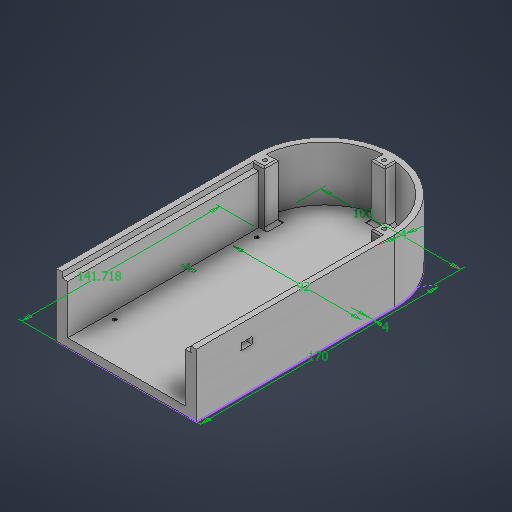
# Autodesk Inventor part: BASE_MANIPULADOR
Saved by Autodesk Inventor 2027.1 (Build 311270010, 270A)
## iProperties
Created: 2026-08-16
Part Number: BASE_MANIPULADOR
Material: Genérico
Document SubType Name: Modeling
Designer: Evellyn
Density: 1 g/cm^3
Appearance: Padrão
Author: Evellyn
Autodesk Inventor part; units mm, degrees
ref_plane "YZ Plane" through (0, 0, 0) normal (1, 0, 0) x (0, 1, 0)
ref_plane "XZ Plane" through (0, 0, 0) normal (0, 1, 0) x (-1, 0, 0)
ref_plane "XY Plane" through (0, 0, 0) normal (0, 0, 1) x (1, 0, 0)
sketch "Esboço1" plane through (0, 0, 0) normal (0, 1, 0) x (-1, 0, 0)
  point P0 (0, 0)
sketch "Esboço2" plane through (0, 0, 0) normal (0, 1, 0) x (-1, 0, 0)
  line L0 (50, -56.7182) -> (50, 85)
  line L1 (50, 85) -> (-50, 85)
  line L2 (-50, 85) -> (-50, -56.7182)
  line L3 (-50, -85) -> (50, 85) construction
  line L4 (50, -85) -> (-50, 85) construction
  line L5 (50, 0) -> (-50, 0)
  line L6 (-50, 0) -> (-50, -56.7182)
  line L7 (50, -56.7182) -> (50, 0)
  line L8 (0, 0) -> (0, -6.7182)
  arc A0 (-50, -56.7182) -> (50, -56.7182) centre (0, -56.7182) ccw
  line L9 (46, 85) -> (46, -56.7182)
  line L10 (-46, 85.0696) -> (-46, -56.7182)
  arc A1 (-46, -56.7182) -> (46, -56.7182) centre (0, -56.7182) ccw
  point P0 (-46, 85)
  dimension "d0" = 170
  dimension "d1" = 100
  dimension "d2" = 4
  dimension "d64" = 141.7182
  dimension "d70" = 4
  dimension "d71" = 4
  dimension "d72" = 92
  constraints: 22 end point, 5 point on circle, 3 point on line, 2 centre point, 2 midpoint, 2 parallel, 1 concentric, 1 horizontal, 1 perpendicular, 1 tangent, 1 vertical
  measures "d0" distance of L1.end L3.start
  measures "d1" distance of L3.start L4.start
  measures "d2" distance between parallel lines of L9 L0
  measures "d64" distance of L0.start L0.end
  measures "d70" distance between parallel lines of L6 L10
  measures "d71" radial gap between concentric circles of A1 A0
  measures "d72" distance between parallel lines of L10 L9
extrude "Extrusão3" add sketch "Esboço2" along normal blind 6 contours L9 A1 L10 L5 | L5 L10 L1 L9
extrude "Extrusão4" add sketch "Esboço2" along normal blind 45 contours A0 L2 L5 L10 A1 L9 L0 | L5 L9 L1 L0 | L2 L1 L10 L5
sketch "Esboço3" plane through (0, 6, 0) normal (0, 1, 0) x (1, 0, 0)
  line L0 (-37.999, -80.9605) -> (38.001, -80.9605)
  line L1 (40.001, -78.9605) -> (40.001, 62.0395)
  line L2 (38.001, 64.0395) -> (-37.999, 64.0395)
  line L3 (-39.999, 62.0395) -> (-39.999, -78.9605)
  line L4 (-46, -85) -> (-46, 56.7182) projected
  arc A0 (-39.999, -78.9605) -> (-37.999, -80.9605) centre (-37.999, -78.9605) ccw
  arc A1 (-37.999, 64.0395) -> (-39.999, 62.0395) centre (-37.999, 62.0395) ccw
  arc A2 (-37.999, 64.0395) -> (-39.999, 62.0395) centre (-37.999, 62.0395) ccw
  arc A3 (38.001, -80.9605) -> (40.001, -78.9605) centre (38.001, -78.9605) ccw
  circle A4 centre (-36.649, -56.8397) radius 1.35
  circle A5 centre (36.651, -56.7985) radius 1.35
  circle A6 centre (-36.649, 44.8205) radius 1.35
  circle A7 centre (36.651, 44.8205) radius 1.35
  arc A8 (40.001, 62.0395) -> (38.001, 64.0395) centre (38.001, 62.0395) ccw
  point P0 (0, 0)
  point P1 (40.001, 64.0395)
  point P2 (40.001, -80.9605)
  point P3 (-39.999, 64.0395)
  dimension "d11" = 80
  dimension "d12" = 145
  dimension "d13" = 6.001
  dimension "d14" = 2
  dimension "d15" = 2.7
  dimension "d17" = 3.35
  dimension "d18" = 2.7
  dimension "d19" = 3.35
  dimension "d20" = 22.162
  dimension "d21" = 2.7
  dimension "d22" = 3.35
  dimension "d23" = 17.219
  dimension "d24" = 2.7
  dimension "d25" = 3.35
  dimension "d26" = 2
  dimension "d27" = 17.219
  constraints: 10 point on circle, 10 tangent, 9 centre point, 8 end point, 8 point on line, 3 equal radius, 2 parallel, 1 horizontal, 1 perpendicular
  measures "d11" distance of point (-39.999, 64.039) point (40.001, 64.039)
  measures "d12" distance of point (40.001, 64.039) point (40.001, -80.961)
  measures "d13" distance between parallel lines of L4 L3
  measures "d14" radius of A0
  measures "d15" diameter of A4
  measures "d17" distance from line of L3 A4.centre
  measures "d18" diameter of A5
  measures "d19" distance from line of L1 A5.centre
  measures "d20" vertical distance of A5.centre A3.centre
  measures "d21" diameter of A6
  measures "d22" distance from line of L3 A6.centre
  measures "d23" vertical distance of A2.centre A6.centre
  measures "d24" diameter of A7
  measures "d25" distance from line of L1 A7.centre
  measures "d26" radius of A8
  measures "d27" vertical distance of A8.centre A7.centre
extrude "Extrusão5" cut sketch "Esboço3" against normal blind 3 contours A4 | A5 | A6 | A7
sketch "Esboço4" plane through (0, 6, 0) normal (0, 1, 0) x (1, 0, 0)
  arc A0 (46, 56.7182) -> (-46, 56.7182) centre (0, 56.7182) ccw projected
  line L0 (-46, -85) -> (-46, 56.7182) projected
  line L1 (46, 56.7182) -> (46, -85) projected
  line L2 (0, 112.992) -> (0, 0)
  line L3 (-5, 94.9519) -> (5, 94.9519)
  line L4 (5, 94.9519) -> (5, 104.9519)
  line L5 (5, 104.9519) -> (-5, 104.9519)
  line L6 (-5, 104.9519) -> (-5, 94.9519)
  line L7 (-5, 94.9519) -> (5, 104.9519) construction
  line L8 (5, 94.9519) -> (-5, 104.9519) construction
  circle A1 centre (0, 56.7182) radius 48.2336
  arc A2 (50, 56.7182) -> (-50, 56.7182) centre (0, 56.7182) ccw projected
  line L9 (-51.2088, 56.7182) -> (50, 56.7182)
  line L10 (48.2336, 61.7182) -> (38.2336, 61.7182)
  line L11 (38.2336, 51.7182) -> (48.2336, 51.7182)
  line L12 (48.2336, 51.7182) -> (48.2336, 61.7182)
  line L13 (38.2336, 61.7182) -> (38.2336, 51.7182)
  line L14 (-48.2336, 51.7182) -> (-38.2336, 51.7182)
  line L15 (-38.2336, 61.7182) -> (-48.2336, 61.7182)
  line L16 (-48.2336, 61.7182) -> (-48.2336, 51.7182)
  line L17 (-38.2336, 51.7182) -> (-38.2336, 61.7182)
  point P0 (0, 99.9519)
  point P1 (46, 51.7182)
  point P2 (45.7275, 61.7182)
  point P3 (-45.7275, 61.7182)
  point P4 (-46, 51.7182)
  point P5 (5, 102.4457)
  point P6 (-5, 102.4457)
  dimension "d30" = 10
  dimension "d31" = 10
  dimension "d34" = 180
  dimension "d65" = 96.4673
  constraints: 32 end point, 2 horizontal, 2 midpoint, 2 parallel, 1 centre point, 1 coincident, 1 perpendicular, 1 point on line, 1 tangent, 1 vertical, 17 other
  measures "d30" distance of L5.end L4.end
  measures "d31" distance of L4.end L3.end
  measures "d65" diameter of A1
extrude "Extrusão6" add sketch "Esboço4" along normal blind 39 contours L9 L13 L10 A0 | L1 L11 L13 L9 | L4 L3 L2 A0 | L2 L3 L6 A0 | L17 L14 L0 L9 | L9 A0 L15 L17
fillet "Arredondamento da face2" radius 2 1 edges at (0, 6, -94.9519)
fillet "Arredondamento da face4" radius 2 1 edges at (-38.2336, 6, -56.7182)
fillet "Arredondamento da face5" radius 2 1 edges at (-41.9805, 6, -61.7182)
fillet "Arredondamento da face6" radius 2 1 edges at (-5, 6, -98.6988)
fillet "Arredondamento da face7" radius 2 1 edges at (38.2336, 6, -56.7182)
fillet "Arredondamento da face8" radius 2 1 edges at (5, 6, -98.6988)
fillet "Arredondamento da face9" radius 3 1 edges at (41.9805, 6, -61.7182)
fillet "Arredondamento1" radius 1 9 edges at (-42.1168, 45, -51.7182) (-41.9805, 45, -61.7182) (-38.2336, 45, -56.7182) (0, 45, -94.9519) (-5, 45, -98.6988) (5, 45, -98.6988) (41.9805, 45, -61.7182) (38.2336, 45, -56.7182) (42.1168, 45, -51.7182)
sketch "Esboço5" plane through (0, 6, 0) normal (0, 1, 0) x (1, 0, 0)
  line L0 (-50, -85) -> (50, -85) projected
  line L1 (-42, -85) -> (-42, 51.6379)
  line L2 (-46, -85) -> (-46, 52.7182) projected
  line L3 (-36.2336, 51.7182) -> (-46, 51.7182) projected
  line L4 (-42, 51.6379) -> (-42, 51.7182)
  line L5 (42, 51.6379) -> (42, 51.7182)
  line L6 (42, -85) -> (42, 51.7182)
  line L7 (46, 51.7182) -> (36.2336, 51.7182) projected
  line L8 (46, -85) -> (46, 51.7182) projected
  point P0 (0, 0)
  dimension "d48" = 4
  dimension "d49" = 4
  constraints: 8 end point, 3 point on line, 2 vertical, 1 perpendicular
  measures "d48" distance between parallel lines of L1 L2
  measures "d49" distance between parallel lines of L8 L6
extrude "Extrusão7" add sketch "Esboço5" along normal blind 35
sketch "Esboço6" plane through (0, 45, 0) normal (0, 1, 0) x (1, 0, 0)
  arc A0 (-4, 102.544) -> (-45.8258, 60.7182) centre (0, 56.7182) ccw projected
  arc A1 (45.8258, 60.7182) -> (4, 102.544) centre (0, 56.7182) ccw projected
  circle A2 centre (0, 56.7182) radius 46.0304
  line L0 (4, 102.544) -> (4, 95.9519) projected
  line L1 (4, 95.9519) -> (-4, 95.9519) projected
  line L2 (-4, 95.9519) -> (-4, 102.544) projected
  circle A3 centre (0, 56.7182) radius 42.5494
  circle A4 centre (0, 99.2676) radius 1.35
  circle A5 centre (42.5494, 56.7182) radius 1.35
  circle A6 centre (-42.5494, 56.7182) radius 1.35
  point P0 (0, 0)
  dimension "d52" = 2.7
  dimension "d55" = 180
  constraints: 4 centre point, 2 coincident, 1 vertical alignment, 7 other
  measures "d52" diameter of A4
extrude "Extrusão8" cut sketch "Esboço6" against normal blind 8 contours A5 A3 | A3 A5 | A4 A3 | A3 A4 | A6 A3 | A3 A6
sketch "Esboço7" plane through (0, 41, 0) normal (0, 1, 0) x (1, 0, 0)
  circle A0 centre (44, -45) radius 1.35
  line L0 (42, 51.7182) -> (42, -85) projected
  line L1 (46, 52.7182) -> (46, -85) projected
  line L2 (42, -85) -> (46, -85) projected
  point P0 (0, 0)
  point P1 (44, -85)
  dimension "d59" = 2.7
  dimension "d60" = 40
  dimension "d61" = 2
  constraints: 1 centre point, 1 midpoint
  measures "d59" diameter of A0
  measures "d60" distance of point (44, -85) A0.centre
  measures "d61" distance from line of L0 A0.centre
extrude "Extrusão9" cut sketch "Esboço7" against normal blind 8
sketch "Esboço8" plane through (50, 0, 85) normal (1, 0, 0) x (0, 0, -1)
  line L0 (31.9145, 32.9132) -> (39.7145, 32.9132)
  line L1 (39.7145, 32.9132) -> (39.7145, 28.2132)
  line L2 (39.7145, 28.2132) -> (31.9145, 28.2132)
  line L3 (31.9145, 28.2132) -> (31.9145, 32.9132)
  point P0 (85, 0)
  dimension "d66" = 7.8
  dimension "d67" = 4.7
  constraints: 8 end point, 2 parallel, 1 horizontal, 1 perpendicular
  measures "d66" distance of L1.end L2.end
  measures "d67" distance of L0.end L1.end
extrude "Extrusão10" cut sketch "Esboço8" against normal blind 10
